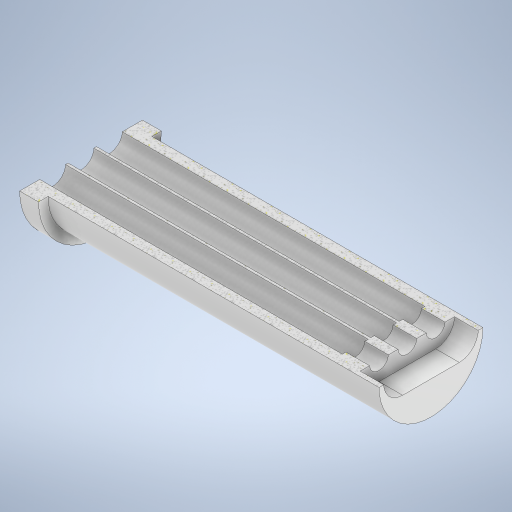
# Autodesk Inventor part: 029
Saved by Autodesk Inventor 2023 (Build 270158000, 158)
## iProperties
Created: 2022-04-04
Part Number: 029
Material: Acetal Resin, White
Document SubType Name: Modeling
Designer: Vinicius Miguel
Density: 1.425 g/cm^3
Appearance: Smooth - White
Mass: 23.4979 g
Surface Area: 85.2942 cm^2
Volume: 16.4897 cm^3
Author: Vinicius Miguel
Autodesk Inventor part; units mm, degrees
ref_plane "YZ Plane" through (0, 0, 0) normal (1, 0, 0) x (0, 1, 0)
ref_plane "XZ Plane" through (0, 0, 0) normal (0, 1, 0) x (-1, 0, 0)
ref_plane "XY Plane" through (0, 0, 0) normal (0, 0, 1) x (1, 0, 0)
sketch "Sketch1" plane through (0, 0, 0) normal (0, 1, 0) x (-1, 0, 0)
  line L0 (0, 0) -> (74, 0)
  line L1 (74, 0) -> (74, -13)
  line L2 (74, -13) -> (70, -13)
  line L3 (70, -13) -> (70, -11)
  line L4 (70, -11) -> (0, -11)
  line L5 (0, -11) -> (0, 0)
  dimension "d0" = 22
  dimension "d1" = 70
  dimension "d2" = 26
  dimension "d3" = 4
  constraints: 12 end point, 5 perpendicular, 1 horizontal
  measures "d0" diameter of L4 L0
  measures "d1" distance of L3.end L4.end
  measures "d2" diameter of L2 L0
  measures "d3" distance of L1.end L2.end
revolve "Revolution1" add sketch "Sketch1" angle 360 about axis through (0, 0, 0) along (-1, 0, 0)
sketch "Sketch3" plane through (0, 0, 0) normal (0, 1, 0) x (-1, 0, 0)
  line L0 (0, 0) -> (74, 0)
  line L1 (74, 13) -> (74, -13) projected
  line L2 (0, 0) -> (0, 4)
  line L3 (0, 11) -> (0, -11) projected
  line L4 (0, 4) -> (5, 4)
  line L5 (5, 4) -> (5, 2)
  line L6 (5, 2) -> (10, 2)
  line L7 (10, 2) -> (10, 2.75)
  line L8 (10, 2.75) -> (74, 2.75)
  dimension "d16" = 5.5
  dimension "d17" = 8
  dimension "d18" = 4
  dimension "d19" = 5
  dimension "d20" = 5
  constraints: 14 end point, 4 perpendicular, 2 horizontal, 2 point on line, 1 midpoint
  measures "d16" diameter of L8 L0
  measures "d17" diameter of L4 L0
  measures "d18" diameter of L6 L0
  measures "d19" distance of L2.end L4.end
  measures "d20" distance of L5.end L6.end
revolve "Revolution2" cut sketch "Sketch3" angle 360 about axis through (0, 0, 0) along (-1, 0, 0)
pattern_linear "Rectangular Pattern1" count 2 spacing 6 along (0, 0, 1) of "Revolution2"
pattern_linear "Rectangular Pattern2" count 2 spacing 6 along (0, 0, -1) of "Revolution2"
sketch "Sketch4" plane through (0, 0, 0) normal (1, 0, 0) x (0, 0, -1)
  arc A0 (-3, 2.6458) -> (-3, -2.6458) centre (-6, 0) ccw construction
  arc A1 (3, -2.6458) -> (3, 2.6458) centre (6, 0) ccw construction
  circle A2 centre (-6, 0) radius 2 projected
  circle A3 centre (6, 0) radius 2 projected
  line L0 (-6, 0) -> (6, 0) construction
  line L1 (-6, -4) -> (6, -4)
  line L2 (6, 4) -> (-6, 4)
  arc A4 (-6, 4) -> (-6, -4) centre (-6, 0) ccw
  arc A5 (6, -4) -> (6, 4) centre (6, 0) ccw
  point P0 (0, 0)
  point P1 (0, 0)
  constraints: 8 end point, 4 point on circle, 4 tangent, 2 centre point, 1 concentric, 1 midpoint, 1 parallel
extrude "Extrusion1" cut sketch "Sketch4" against normal up to surface (5 mm away) contours A2 | A3 | A4 L2 A5 L1
body "Solid1"
